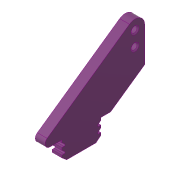
# Autodesk Inventor part: control_horn
Saved by Autodesk Inventor 2019 (Build 230136000, 136)
## iProperties
Created: 2022-04-02
Part Number: control_horn
Material: ABS Plastic
Document SubType Name: Modeling
Designer: solyo
Density: 1.06 g/cm^3
Appearance: Smooth - Purple
Mass: 0.390386 g
Surface Area: 5.14036 cm^2
Volume: 0.368289 cm^3
Author: solyo
Autodesk Inventor part; units mm, degrees
ref_plane "YZ Plane" through (0, 0, 0) normal (1, 0, 0) x (0, 1, 0)
ref_plane "XZ Plane" through (0, 0, 0) normal (0, 1, 0) x (-1, 0, 0)
ref_plane "XY Plane" through (0, 0, 0) normal (0, 0, 1) x (1, 0, 0)
sketch "Sketch1" plane through (0, 0, 0) normal (1, 0, 0) x (0, 1, 0)
  line L0 (0, 0) -> (13.6383, -19.4775)
  line L1 (12, -22.6247) -> (4.9015, -22.6247)
  line L2 (0, -15.6247) -> (4.9015, -22.6247)
  line L3 (0, 0) -> (0, -5.6247)
  line L4 (0, -5.6247) -> (-4, -5.6247)
  line L5 (-4, -5.6247) -> (-4, -13.6247)
  line L6 (-4, -13.6247) -> (0, -13.6247)
  line L7 (0, -13.6247) -> (0, -15.6247)
  arc A0 (12, -22.6247) -> (13.6383, -19.4775) centre (12, -20.6247) ccw
  point P0 (15.842, -22.6247)
  point P1 (9, -20.6247)
  dimension "d26" = 8
  dimension "d31" = 4
  dimension "d32" = 2
  dimension "d43" = 2
  dimension "d44" = 5
  dimension "d45" = 12
  dimension "d56" = 35
  dimension "d64" = 3
  constraints: 16 end point, 3 parallel, 3 point on line, 2 horizontal, 2 point on circle, 2 tangent, 1 centre point, 1 coincident, 1 collinear, 1 vertical
  measures "d26" distance of L4.end L5.end
  measures "d31" distance between parallel lines of L3 L5
  measures "d32" distance of L6.end L2.start
  measures "d43" radius of A0
  measures "d44" vertical distance of L2.start A0.centre
  measures "d45" horizontal distance of L0.start point (12, -20.625)
  measures "d56" angle of L3 L0
  measures "d64" distance of A0.centre point (9, -20.625)
extrude "Extrusion1" add sketch "Sketch1" along normal blind 2
hole "Hole3" at (0, 12, -20.6247) at (0, 9, -20.6247) direction (1, 0, 0) diameter 1.2 end through all
fillet "Fillet3" radius 1 1 edges at (1, 0, 0)
chamfer "Chamfer2" distance 0.2 angle 45 4 edges at (2, 12, -21.2247) (0, 12, -21.2247) (0, 9, -21.2247) (2, 9, -21.2247)
ref_plane "Work Plane1" through (0, -4, -9.6247) normal (0, 0, -1) x (-1, 0, 0)
sketch "Sketch4" plane through (2, 0, 0) normal (1, 0, 0) x (0, 0, -1)
  arc A0 (2.598, 1.8192) -> (3.1716, 0) centre (3.1716, 1) ccw projected
  line L0 (3.1716, 0) -> (5.6247, 0) projected
  line L1 (5.6247, 0) -> (5.6247, -4) projected
  line L2 (5.6247, -4) -> (13.6247, -4) projected
  line L3 (13.6247, -4) -> (13.6247, 0) projected
  line L4 (13.6247, 0) -> (15.6247, 0) projected
  line L5 (15.6247, 0) -> (22.6247, 4.9015) projected
  line L6 (22.6247, 4.9015) -> (22.6247, 12) projected
  arc A1 (22.6247, 12) -> (19.4775, 13.6383) centre (20.6247, 12) ccw projected
  line L7 (19.4775, 13.6383) -> (2.598, 1.8192) projected
  circle A2 centre (20.6247, 12) radius 0.8 projected
  line L8 (5.6247, 0) -> (13.6247, 0)
  line L9 (13.6247, -4) -> (5.6247, -4) projected
  line L10 (6.6247, -4) -> (5.6247, -3.1667)
  line L11 (5.6247, -4) -> (5.6247, 0) projected
  line L12 (5.6247, -2.6667) -> (6.6247, -2.6667)
  line L13 (6.6247, -2.6667) -> (5.6247, -1.8333)
  line L14 (5.6247, -1.3333) -> (6.6247, -1.3333)
  line L15 (6.6247, -1.3333) -> (5.6247, -0.5)
  line L16 (5.6247, -0.5) -> (5.6247, 0)
  line L17 (5.6247, -0.5) -> (5.6247, -1.3333)
  line L18 (5.6247, -1.8333) -> (5.6247, -2.6667)
  line L19 (5.6247, -3.1667) -> (5.6247, -4)
  line L20 (5.6247, -4) -> (6.6247, -4)
  point P0 (0, 0)
  dimension "d57" = 1
  dimension "d58" = 0.5
  dimension "d59" = 0.5
  dimension "d60" = 0.5
  constraints: 22 end point, 6 point on line, 3 collinear, 3 perpendicular, 2 parallel, 2 vertical alignment, 1 horizontal, 1 vertical
  measures "d57" distance of L1.end L10.start
  measures "d58" distance of L13.end L14.start
  measures "d59" distance of L12.start L10.end
  measures "d60" distance of L15.end L0.end
extrude "Extrusion2" cut sketch "Sketch4" against normal through all contours L15 L14 L1 | L13 L12 L1 | L2 L1 L10
mirror "Mirror1" about plane through (0, -4, -9.6247) normal (0, 0, -1) of "Extrusion2"
fillet "Fillet4" radius 0.2 4 edges at (1, -1.3333, -12.6247) (1, -2.6667, -12.6247) (1, -1.3333, -6.6247) (1, -2.6667, -6.6247)
equation "\"d59\" = d58"
equation "\"d60\" = d58"
equation "\"d1\" = d0"
equation "\"d21\" = d1"
equation "\"d0\" = 12"
body "Solid1"
